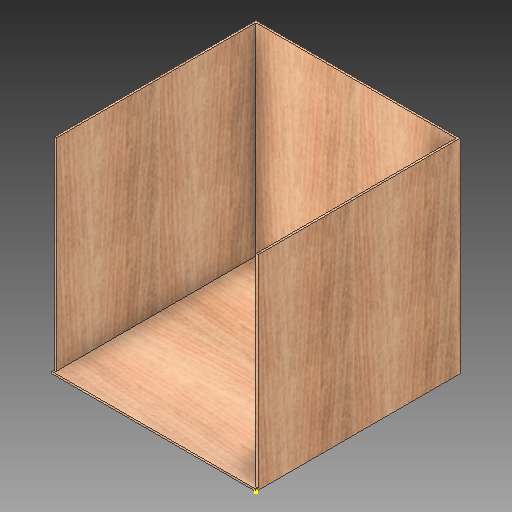
# Autodesk Inventor part: boite
Saved by Autodesk Inventor 2019 (Build 230136000, 136)
## iProperties
Created: 2018-11-20
Part Number: boite
Material: Bois (bouleau)
Document SubType Name: Modeling
Designer: pouey
Density: 0.55 g/cm^3
Appearance: Bouleau - Poli naturel
Author: pouey
Autodesk Inventor part; units mm, degrees
ref_plane "YZ Plane" through (0, 0, 0) normal (1, 0, 0) x (0, 1, 0)
ref_plane "XZ Plane" through (0, 0, 0) normal (0, 1, 0) x (-1, 0, 0)
ref_plane "XY Plane" through (0, 0, 0) normal (0, 0, 1) x (1, 0, 0)
sketch "Esquisse1" plane through (0, 0, 0) normal (0, 1, 0) x (-1, 0, 0)
  point P0 (0, 0)
sketch "Esquisse2" plane through (0, 0, 0) normal (0, 1, 0) x (-1, 0, 0)
  line L0 (0, 0) -> (500, 0)
  line L1 (500, 0) -> (500, -500)
  line L2 (500, -500) -> (0, -500)
  line L3 (0, -500) -> (0, 0)
  dimension "d0" = 500
  dimension "d1" = 500
  constraints: 8 end point, 2 parallel, 1 horizontal, 1 perpendicular
  measures "d0" distance of L0.end L1.end
  measures "d1" distance of L1.end L2.end
sketch "Esquisse3" plane through (0, 0, 0) normal (0, 1, 0) x (-1, 0, 0)
  line L0 (0, 0) -> (500, 0)
  line L1 (500, 0) -> (500, -5)
  line L2 (500, -5) -> (0, -5)
  line L3 (0, -5) -> (0, 0)
  line L4 (500, -5) -> (495, -5)
  line L5 (495, -5) -> (495, -500)
  line L6 (495, -500) -> (500, -500)
  line L7 (500, -500) -> (500, -5)
  line L8 (495, -500) -> (0, -500)
  line L9 (0, -500) -> (0, -495)
  line L10 (0, -495) -> (495, -495)
  line L11 (495, -495) -> (495, -500)
  line L12 (0, -5) -> (5, -5)
  line L13 (5, -5) -> (5, -495)
  line L14 (5, -495) -> (0, -495)
  line L15 (0, -495) -> (0, -5)
  dimension "d2" = 500
  dimension "d3" = 5
  dimension "d4" = 495
  dimension "d5" = 5
  dimension "d6" = 495
  dimension "d7" = 5
  dimension "d8" = 5
  constraints: 32 end point, 8 parallel, 4 horizontal, 4 perpendicular, 1 point on line
  measures "d2" distance of L1.end L2.end
  measures "d3" distance between parallel lines of L0 L2
  measures "d4" distance of L4.end L5.end
  measures "d5" distance between parallel lines of L7 L5
  measures "d6" distance of L9.end L10.end
  measures "d7" distance between parallel lines of L8 L10
  measures "d8" distance between parallel lines of L15 L13
extrude "Extrusion1" add sketch "Esquisse3" along normal blind 500 contours L2 L13 L10 L15 | L7 L6 L5 L2 | L10 L5 L8 L9
extrude "Extrusion2" add sketch "Esquisse2" along normal blind 5
